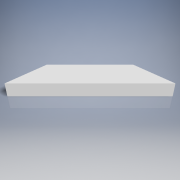
# Autodesk Inventor part: L Support Joist
Saved by Autodesk Inventor 2018 (Build 220112000, 112)
## iProperties
Created: 2018-07-21
Part Number: L Support Joist
Material: Generic
Document SubType Name: Modeling
Designer: jjsch
Density: 1 g/cm^3
Appearance: Default
Author: jjsch
Autodesk Inventor part; units mm, degrees
ref_plane "YZ Plane" through (0, 0, 0) normal (1, 0, 0) x (0, 1, 0)
ref_plane "XZ Plane" through (0, 0, 0) normal (0, 1, 0) x (-1, 0, 0)
ref_plane "XY Plane" through (0, 0, 0) normal (0, 0, 1) x (1, 0, 0)
sketch "Sketch1" plane through (0, 0, 0) normal (0, 1, 0) x (-1, 0, 0)
  line L0 (0, 0) -> (-287.3682, -287.3682)
  line L1 (0, 0) -> (406.4, 0) construction
  line L2 (-287.3682, -287.3682) -> (-350.23, -224.5064)
  line L3 (-350.23, -224.5064) -> (-62.8618, 62.8618)
  line L4 (-62.8618, 62.8618) -> (0, 0)
  line L5 (-62.8618, 62.8618) -> (-62.8618, -62.8618)
  line L6 (-350.23, -224.5064) -> (-224.5064, -224.5064)
  dimension "d0" = 406.4
  dimension "d1" = 135
  dimension "d2" = 88.9
  constraints: 14 end point, 4 perpendicular, 2 point on line, 1 equal length, 1 horizontal, 1 vertical
  measures "d0" distance of L0.start L0.end
  measures "d1" angle of L0 L1
  measures "d2" distance of L0.end L2.end
extrude "Extrusion1" add sketch "Sketch1" along normal blind 38.1 contours L0 L6 L3 L5
body "Solid1"
